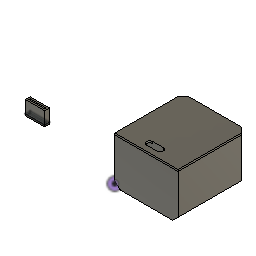
esp-clock-case (Autodesk Fusion 360 design; units mm, degrees)
Autodesk Fusion 360 part; units mm, degrees
note: some values were not read from the file. Chosen so that the rebuilt part matches the saved one: which face or edge a step refers to. Set by a fixed rule: which sketch regions a step uses.
sketch "Screen" plane through (0, 0, 0) normal (0, 0, 1) x (1, 0, 0) in component "Front"
  line L0 (0, 0) -> (36, 0)
  line L1 (36, 0) -> (36, 39)
  line L2 (36, 39) -> (0, 39)
  line L3 (0, 39) -> (0, 0)
  line L4 (5.5, 28.6) -> (30.5, 28.6)
  line L5 (30.5, 28.6) -> (30.5, 10.6)
  line L6 (30.5, 10.6) -> (5.5, 10.6)
  line L7 (5.5, 10.6) -> (5.5, 28.6)
  line L8 (5.5, 14.6) -> (30.5, 14.6)
  line L9 (4, 33.6) -> (32, 33.6)
  line L10 (32, 33.6) -> (32, 4.6)
  line L11 (32, 4.6) -> (4, 4.6)
  line L12 (4, 4.6) -> (4, 33.6)
  line L13 (12, 33.6) -> (12, 28.6)
  line L14 (24, 33.6) -> (24, 28.6)
  line L15 (34.4, 37.4) -> (1.6, 37.4)
  line L16 (1.6, 37.4) -> (1.6, 1.6)
  line L17 (1.6, 1.6) -> (34.4, 1.6)
  line L18 (34.4, 1.6) -> (34.4, 37.4)
  line L19 (12, 29.6) -> (24, 29.6)
  dimension "d1" = 25
  dimension "d2" = 18
  dimension "d4" = 14
  dimension "d5" = 28
  dimension "d6" = 29
  dimension "d7" = 1.5
  dimension "d8" = 1.5
  dimension "d9" = 5
  dimension "d10" = 12
  dimension "d11" = 8
  dimension "d12" = 8
  dimension "d13" = 39
  dimension "d14" = 36
  dimension "d15" = -1.6
  dimension "d16" = 4
  dimension "d17" = 4
  dimension "d81" = 3
  dimension "d105" = 1
  constraint horizontal L0
  constraint vertical L1
  constraint horizontal L2
  constraint vertical L3
  constraint coincident L0.start L3.end
  constraint horizontal L4
  constraint vertical L5
  constraint horizontal L6
  constraint vertical L7
  constraint coincident L7 L8.start
  constraint coincident L5 L8.end
  constraint perpendicular L5 L8
  constraint horizontal L9
  constraint vertical L10
  constraint horizontal L11
  constraint vertical L12
  constraint coincident L9 L13.start
  constraint coincident L4 L13.end
  constraint perpendicular L4 L13
  constraint coincident L9 L14.start
  constraint coincident L4 L14.end
  constraint perpendicular L4 L14
  constraint coincident L13 L19.start
  constraint coincident L14 L19.end
  constraint perpendicular L14 L19
  measures "d1" distance of L4.start L4.end
  measures "d2" distance of L4.start L6.end
  measures "d4" distance of L4 L8
  measures "d5" distance of L9.start L9.end
  measures "d6" distance of L9.start L11.end
  measures "d7" distance of L7 L12
  measures "d8" distance of L5 L10
  measures "d9" distance of L4 L9
  measures "d10" distance of L13 L14
  measures "d11" distance of L10 L14
  measures "d12" distance of L12 L13
  measures "d13" distance of L0 L2
  measures "d14" distance of L1 L3
  measures "d16" distance of L3 L12
  measures "d17" distance of L1 L10
  measures "d81" distance of L11 L17
  measures "d105" distance of L4 L19
extrude "Extrude1" add sketch "Screen" along normal blind 0.2 contours L4 L13 L14 L19 | L5 L6 L7 L8 | L9 L13 L14 L19 makes body 1 at (13.8333, 13.2667, 0) makes body 2 at (16, 30.2667, 0) in component "Front"
extrude "Extrude2" add sketch "Screen" along normal blind 1 contours L4 L5 L6 L7 L9 L10 L11 L12 L13 L14 | L4 L13 L14 L19 bodies 1 2 in component "Front"
extrude "Extrude4" add sketch "Screen" along normal blind 24 contours L0 L1 L2 L3 bodies 1 makes body 3 in component "Front"
sketch "ESP32" plane through (0, 1.6, 0) normal (0, 1, 0) x (-1, 0, 0) in component "Front"
  line L0 (-34.4, 0) -> (-1.6, 0)
  line L1 (-1.6, 0) -> (-1.6, 24)
  line L2 (-1.6, 24) -> (-34.4, 24)
  line L3 (-34.4, 24) -> (-34.4, 0)
  line L4 (-9, 1) -> (-27, 1)
  line L5 (-27, 1) -> (-27, 24)
  line L6 (-27, 24) -> (-9, 24)
  line L7 (-9, 24) -> (-9, 1)
  line L8 (-16, 1) -> (-23, 1)
  line L9 (-23, 1) -> (-23, 4)
  line L10 (-23, 4) -> (-16, 4)
  line L11 (-16, 4) -> (-16, 1)
  line L12 (-11, 1) -> (-14.8, 1)
  line L13 (-14.8, 1) -> (-14.8, 4)
  line L14 (-14.8, 4) -> (-11, 4)
  line L15 (-11, 4) -> (-11, 1)
  line L16 (-11, 24) -> (-11, 1)
  line L17 (-25, 1) -> (-25, 24)
  dimension "d112" = 18
  dimension "d113" = 23
  dimension "d114" = 7.4
  dimension "d115" = 7.4
  dimension "d134" = 7
  dimension "d135" = 4
  dimension "d136" = 3
  dimension "d139" = 2
  dimension "d140" = 12.2
  dimension "d150" = 2
  dimension "d151" = 2
  constraint horizontal L4
  constraint vertical L5
  constraint horizontal L6
  constraint vertical L7
  constraint collinear L2 L6
  constraint horizontal L8
  constraint vertical L9
  constraint horizontal L10
  constraint vertical L11
  constraint coincident L4 L8.start
  constraint horizontal L12
  constraint vertical L13
  constraint horizontal L14
  constraint vertical L15
  constraint coincident L4 L12.start
  constraint collinear L10 L14
  constraint coincident L6 L16.start
  constraint perpendicular L4 L16
  constraint coincident L4 L17.start
  constraint coincident L6 L17.end
  measures "d112" distance of L4.start L4.end
  measures "d113" distance of L4.start L6.end
  measures "d114" distance of L1 L7
  measures "d115" distance of L3 L5
  measures "d134" distance of L7 L11
  measures "d135" distance of L5 L9
  measures "d136" distance of L4 L10
  measures "d139" distance of L7 L15
  measures "d140" distance of L5 L13
  measures "d150" distance of L7 L16
  measures "d151" distance of L5 L17
extrude "Extrude3" add sketch "Screen" along normal blind 2.5 contours L15 L16 L17 L18 bodies 1 in component "Front"
extrude "Extrude15" add sketch "ESP32" along normal blind 2 contours L0 L1 L2 L3 L4 L5 L7 L8 L12 bodies 1 3 in component "Front"
extrude "Extrude18" cut sketch "ESP32" along normal up to surface (3 mm away) contours L4 L12 L13 L14 L15 L16 | L4 L8 L9 L10 L11 bodies 1 in component "Front"
extrude "Extrude16" cut sketch "ESP32" along normal up to surface (2 mm away) contours L2 L4 L5 L6 L17 | L2 L4 L6 L7 L15 L16 | L2 L4 L6 L9 L10 L11 L13 L14 L16 L17 | L4 L12 L13 L14 L15 L16 | L4 L8 L9 L10 L11 bodies 1 in component "Front"
extrude "Extrude5" add sketch "Screen" against normal blind 1.6 contours L0 L1 L2 L3 | L4 L5 L6 L7 L9 L10 L11 L12 L13 L14 | L4 L13 L14 L19 | L5 L6 L7 L8 | L9 L13 L14 L19 | L15 L16 L17 L18 bodies 1 in component "Front"
extrude "Extrude19" cut sketch "ESP32" against normal blind 0.5 contours L2 L4 L5 L6 L17 | L2 L4 L6 L7 L15 L16 bodies 1 in component "Front"
sketch "Luminosity sensor" plane through (0, 37.4, 0) normal (0, -1, 0) x (1, 0, 0) in component "Front"
  line L0 (1.6, 2.5) -> (34.4, 2.5)
  line L1 (34.4, 2.5) -> (34.4, 24)
  line L2 (34.4, 24) -> (1.6, 24)
  line L3 (1.6, 24) -> (1.6, 2.5)
  line L4 (1.6, 5) -> (32.4, 5)
  line L5 (32.4, 5) -> (32.4, 19.5)
  line L6 (32.4, 19.5) -> (1.6, 19.5)
  line L7 (19.9, 14.5) -> (22.4, 14.5)
  line L8 (22.4, 14.5) -> (22.4, 10)
  line L9 (22.4, 10) -> (19.9, 10)
  line L10 (19.9, 10) -> (19.9, 14.5)
  line L11 (25.4, 19.5) -> (25.4, 5)
  line L12 (19.9, 14.5) -> (15.4, 14.5)
  line L13 (15.4, 14.5) -> (15.4, 10)
  line L14 (15.4, 10) -> (19.9, 10)
  line L15 (19.9, 10) -> (19.9, 14.5)
  line L16 (13.4, 19.5) -> (13.4, 5)
  line L17 (11.4, 24) -> (11.4, 2.5)
  line L18 (15.4, 24) -> (15.4, 2.5)
  dimension "d51" = 14.5
  dimension "d54" = 4.5
  dimension "d55" = 2.5
  dimension "d56" = 4.5
  dimension "d58" = 5
  dimension "d59" = 5
  dimension "d60" = 7
  dimension "d84" = 2
  dimension "d106" = 19
  dimension "d107" = 10
  dimension "d108" = 7
  dimension "d122" = 2
  dimension "d123" = 2
  constraint horizontal L4
  constraint vertical L5
  constraint horizontal L6
  constraint coincident L3 L4.start
  constraint horizontal L7
  constraint vertical L8
  constraint horizontal L9
  constraint vertical L10
  constraint coincident L6 L11.start
  constraint coincident L4 L11.end
  constraint perpendicular L4 L11
  constraint horizontal L12
  constraint vertical L13
  constraint horizontal L14
  constraint vertical L15
  constraint collinear L9 L14
  constraint coincident L6 L16.start
  constraint coincident L4 L16.end
  constraint perpendicular L4 L16
  constraint coincident L2 L17.start
  constraint coincident L0 L17.end
  constraint perpendicular L0 L17
  constraint coincident L2 L18.start
  constraint coincident L0 L18.end
  constraint perpendicular L0 L18
  constraint collinear L13 L18
  measures "d51" distance of L4 L6
  measures "d54" distance of L2 L6
  measures "d55" distance of L7.start L7.end
  measures "d56" distance of L7.start L9.end
  measures "d58" distance of L6 L7
  measures "d59" distance of L4 L9
  measures "d60" distance of L5 L11
  measures "d84" distance of L1 L5
  measures "d106" distance of L5 L16
  measures "d107" distance of L5 L8
  measures "d108" distance of L8 L13
  measures "d122" distance of L16 L18
  measures "d123" distance of L16 L17
extrude "Extrude9" cut sketch "Luminosity sensor" against normal blind 1 contours L4 L5 L6 L11 | L10 L12 L13 L14 L15 L18 bodies 1 in component "Front"
extrude "Extrude10" cut sketch "Luminosity sensor" against normal up to surface (1.6 mm away) draft 20 contours L7 L8 L9 L10 L15 bodies 1 in component "Front"
extrude "Extrude12" add sketch "Luminosity sensor" along normal blind 2 contours L0 L3 L4 L17 | L0 L4 L17 L18 | L3 L4 L6 L17 | L0 L1 L2 L4 L5 L6 L18 | L4 L6 L16 L17 | L2 L3 L6 L17 | L2 L6 L17 L18 bodies 1 in component "Front"
extrude "Extrude17" add sketch "Luminosity sensor" along normal up to surface (1.8 mm away) from surface at 2 contours L0 L4 L17 L18 | L4 L6 L16 L17 | L4 L6 L13 L16 L18 | L2 L6 L17 L18 bodies 1 in component "Front"
chamfer "Chamfer4" distance 3 angle 45 5 edges at (0, 39, 11.2) (36, 39, 11.2) (18, 39, -1.6) (0, 19.5, -1.6) (36, 19.5, -1.6) on bodies 1 in component "Front"
chamfer "Chamfer4" distance 1.5 angle 45 4 edges at (1.6, 35.4, 13.25) (34.4, 35.4, 13.25) (34.4, 3.6, 13.25) (1.6, 3.6, 13.25) on bodies 1 in component "Front"
sketch "Back" plane through (0, 0, 24) normal (0, 0, 1) x (-1, 0, 0) in component "Back"
  line L0 (-33, -39) -> (-3, -39)
  line L1 (0, -36) -> (0, 0)
  line L2 (0, 0) -> (-36, 0)
  line L3 (-36, 0) -> (-36, -36)
  line L4 (-34.4, -33.9) -> (-34.4, -5.1)
  line L5 (-1.6, -5.1) -> (-1.6, -33.9)
  line L6 (-3.1, -35.4) -> (-11.4, -35.4)
  line L7 (-36, -36) -> (-33, -39)
  line L8 (-3, -39) -> (0, -36)
  line L9 (-34.4, -5.1) -> (-32.9, -3.6)
  line L10 (-32.9, -3.6) -> (-27, -3.6)
  line L11 (-27, -3.6) -> (-27, -1.1)
  line L12 (-25, -1.6) -> (-11, -1.6)
  line L13 (-9, -1.1) -> (-9, -3.6)
  line L14 (-9, -3.6) -> (-3.1, -3.6)
  line L15 (-3.1, -3.6) -> (-1.6, -5.1)
  line L16 (-1.6, -33.9) -> (-3.1, -35.4)
  line L17 (-11.4, -35.4) -> (-11.4, -33.6)
  line L18 (-11.4, -33.6) -> (-15.4, -33.6)
  line L19 (-15.4, -33.6) -> (-15.4, -35.4)
  line L20 (-15.4, -35.4) -> (-32.9, -35.4)
  line L21 (-32.9, -35.4) -> (-34.4, -33.9)
  line L22 (-9, -3.6) -> (-9, -6.6)
  line L23 (-9, -6.6) -> (-27, -6.6)
  line L24 (-27, -3.6) -> (-27, -6.6)
  line L25 (-13.25, -6.6) -> (-22.75, -6.6)
  line L26 (-22.75, -6.6) -> (-22.75, -3.1)
  line L27 (-22.75, -3.1) -> (-13.25, -3.1)
  line L28 (-13.25, -3.1) -> (-13.25, -6.6)
  line L29 (-27, -1.1) -> (-25, -1.1)
  line L30 (-25, -1.1) -> (-25, -1.6)
  line L31 (-11, -1.6) -> (-11, -1.1)
  line L32 (-11, -1.1) -> (-9, -1.1)
  line L33 (-1.7, -5.1414) -> (-1.7, -33.8586)
  line L34 (-1.7, -33.8586) -> (-3.1414, -35.3)
  line L35 (-3.1414, -35.3) -> (-11.3, -35.3)
  line L36 (-11.3, -35.3) -> (-11.3, -33.5)
  line L37 (-11.3, -33.5) -> (-15.5, -33.5)
  line L38 (-15.5, -33.5) -> (-15.5, -35.3)
  line L39 (-15.5, -35.3) -> (-32.8586, -35.3)
  line L40 (-32.8586, -35.3) -> (-34.3, -33.8586)
  line L41 (-34.3, -33.8586) -> (-34.3, -5.1414)
  line L42 (-34.3, -5.1414) -> (-32.8586, -3.7)
  line L43 (-32.8586, -3.7) -> (-26.9, -3.7)
  line L44 (-26.9, -3.7) -> (-26.9, -1.2)
  line L45 (-26.9, -1.2) -> (-25.1, -1.2)
  line L46 (-25.1, -1.2) -> (-25.1, -1.7)
  line L47 (-25.1, -1.7) -> (-10.9, -1.7)
  line L48 (-10.9, -1.7) -> (-10.9, -1.2)
  line L49 (-10.9, -1.2) -> (-9.1, -1.2)
  line L50 (-9.1, -1.2) -> (-9.1, -3.7)
  line L51 (-9.1, -3.7) -> (-3.1414, -3.7)
  line L52 (-3.1414, -3.7) -> (-1.7, -5.1414)
  line L53 (-12, -31.5) -> (-24, -31.5)
  line L54 (-24, -31.5) -> (-24, -24.5)
  line L55 (-24, -24.5) -> (-12, -24.5)
  line L56 (-12, -24.5) -> (-12, -31.5)
  line L57 (-12, -33.6) -> (-12, -29.6)
  line L58 (-24, -33.6) -> (-24, -29.6)
  dimension "d91" = 0.1
  dimension "d127" = 5
  dimension "d128" = 3.5
  dimension "d129" = 9.5
  dimension "d130" = 4.25
  dimension "d131" = 4.25
  dimension "d154" = 2
  dimension "d155" = 7
  constraint coincident L13.end L14.start
  constraint perpendicular L22 L51
  constraint perpendicular L13 L23
  constraint coincident L10.end L11.start
  constraint perpendicular L24 L43
  constraint coincident L23.end L24.end
  constraint horizontal L25
  constraint vertical L26
  constraint horizontal L27
  constraint vertical L28
  constraint collinear L23 L25
  constraint horizontal L53
  constraint vertical L54
  constraint horizontal L55
  constraint vertical L56
  constraint collinear L54 L58
  measures "d127" distance of L12 L23
  measures "d128" distance of L25 L27
  measures "d129" distance of L26 L28
  measures "d130" distance of L22 L28
  measures "d131" distance of L24 L26
  measures "d154" distance of L37 L53
  measures "d155" distance of L53 L55
extrude "Extrude1'" add sketch "Back" along normal blind 1 separate body contours L0 L1 L2 L3 L7 L8 | L4 L9 L10 L18 L19 L20 L21 L24 L37 L38 L39 L40 L41 L42 L43 L57 | L11 L12 L13 L22 L24 L29 L30 L31 L32 L43 L44 L45 L46 L47 L48 L49 L50 L51 | L22 L23 L24 L26 L27 L28 L43 L44 L45 L46 L47 L48 L49 L50 L51 | L22 L23 L24 L25 L33 L34 L35 L36 L37 L38 L39 L40 L41 L42 L43 L51 L52 | L5 L6 L14 L15 L16 L17 L18 L22 L33 L34 L35 L36 L37 L51 L52 L57 | L53 L54 L55 L56 L57 L58 makes body 4 in component "Back"
extrude "Extrude2'" add sketch "Back" against normal blind 2.5 contours L22 L23 L24 L25 L33 L34 L35 L36 L37 L38 L39 L40 L41 L42 L43 L51 L52 bodies 4 in component "Back"
fillet "Fillet1" radius 1.75 4 edges at (13.25, 6.6, 24.5) (22.75, 6.6, 24.5) (22.75, 3.1, 24.5) (13.25, 3.1, 24.5) on bodies 4 in component "Back"
sketch "Protection" plane through (0, 0, 0) normal (0, 0, 1) x (1, 0, 0) in component "Protection"
  line L0 (-59, 10.75) -> (-50, 10.75)
  line L1 (-50, 10.75) -> (-50, 10)
  line L2 (-50, 10) -> (-59, 10)
  line L3 (-59, 10) -> (-59, 10.75)
  line L4 (-60, 11.75) -> (-49, 11.75)
  line L5 (-49, 11.75) -> (-49, 9)
  line L6 (-49, 9) -> (-60, 9)
  line L7 (-60, 9) -> (-60, 11.75)
  dimension "d141" = 9
  dimension "d142" = 0.75
  dimension "d143" = 10
  dimension "d144" = 50
  dimension "d145" = -1
  constraint horizontal L0
  constraint vertical L1
  constraint horizontal L2
  constraint vertical L3
  measures "d141" distance of L0.start L0.end
  measures "d142" distance of L0.start L2.end
  measures "d143" distance of origin L2
  measures "d144" distance of origin L1
extrude "Extrude1''" add sketch "Protection" against normal blind 1 separate body contours L0 L1 L2 L3 | L4 L5 L6 L7 makes body 5 in component "Protection"
extrude "Extrude2''" add sketch "Protection" along normal blind 7 bodies 5 in component "Protection"
component "Front" placed x (1, 0, 0) y (0, 1, 0) z (0, 0, 1) at (0, 0, 0)
component "Back" placed x (1, 0, 0) y (0, 1, 0) z (0, 0, 1) at (0, 0, 0)
component "Protection" placed x (1, 0, 0) y (0, 1, 0) z (0, 0, 1) at (0, 0, 0)
equation "d7 = d8"
equation "d12 = d11"
equation "d16 = d17"
equation "d53 = 4.5 mm"
equation "d54 = d53"
equation "d58 = d59"
equation "d114 = d115"
equation "d123 = d122"
equation "d130 = d131"
equation "d133 = d128 / 2"
named bodies: "Front", "Back", "Cache"
